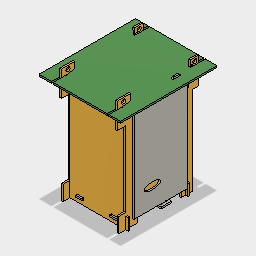
shelter2018-03 (Autodesk Fusion 360 design; units mm, degrees)
Autodesk Fusion 360 part; units mm, degrees
note: some values were not read from the file. Chosen so that the rebuilt part matches the saved one: which face or edge a step refers to. Set by a fixed rule: which sketch regions a step uses.
(part 1 of 2)
sketch "Sketch1" plane through (0, 0, 0) normal (0, 1, 0) x (1, 0, 0)
sketch "Sketch2" plane through (0, 0, 0) normal (0, 1, 0) x (1, 0, 0)
  line L0 (-64.6444, 10.108) -> (17.9056, 10.108)
  line L1 (17.9056, 10.108) -> (17.9056, -78.792)
  line L2 (17.9056, -78.792) -> (-57.0244, -78.792)
  line L3 (-64.6444, -71.172) -> (-64.6444, 10.108)
  line L4 (-53.4684, -78.792) -> (-43.3084, -78.792)
  line L5 (-43.3084, -78.792) -> (-43.3084, -83.872)
  line L6 (-43.3084, -83.872) -> (-53.4684, -83.872)
  line L7 (-53.4684, -83.872) -> (-53.4684, -78.792)
  line L8 (-1.3984, -78.792) -> (10.7936, -78.792)
  line L9 (10.7936, -78.792) -> (10.7936, -83.872)
  line L10 (10.7936, -83.872) -> (-1.3984, -83.872)
  line L11 (-1.3984, -83.872) -> (-1.3984, -78.792)
  line L12 (-49.4044, 10.108) -> (-39.2444, 10.108)
  line L13 (-39.2444, 10.108) -> (-39.2444, 15.188)
  line L14 (-39.2444, 15.188) -> (-49.4044, 15.188)
  line L15 (-49.4044, 15.188) -> (-49.4044, 10.108)
  line L16 (-3.4304, 10.108) -> (9.7776, 10.108)
  line L17 (9.7776, 10.108) -> (9.7776, 15.188)
  line L18 (9.7776, 15.188) -> (-3.4304, 15.188)
  line L19 (-3.4304, 15.188) -> (-3.4304, 10.108)
  line L20 (17.9056, -18.467) -> (27.6846, -18.467)
  line L21 (27.6846, -18.467) -> (27.6846, -34.215)
  line L22 (27.6846, -34.215) -> (17.9056, -34.215)
  line L23 (17.9056, -34.215) -> (17.9056, -18.467)
  line L24 (20.6996, -22.785) -> (23.8746, -22.785)
  line L25 (23.8746, -22.785) -> (23.8746, -29.897)
  line L26 (23.8746, -29.897) -> (20.6996, -29.897)
  line L27 (20.6996, -29.897) -> (20.6996, -22.785)
  line L28 (-56.5164, -21.642) -> (-45.3404, -21.642)
  line L29 (-45.3404, -21.642) -> (-45.3404, -24.182)
  line L30 (-45.3404, -24.182) -> (-56.5164, -24.182)
  line L31 (-56.5164, -24.182) -> (-56.5164, -21.642)
  line L32 (-20.7024, -21.642) -> (-12.5744, -21.642)
  line L33 (-12.5744, -21.642) -> (-12.5744, -24.182)
  line L34 (-12.5744, -24.182) -> (-20.7024, -24.182)
  line L35 (-20.7024, -24.182) -> (-20.7024, -21.642)
  arc A0 (-64.6444, -71.172) -> (-57.0244, -78.792) centre (-57.0244, -71.172) ccw
  line L36 (-2.54, 5.08) -> (12.7, 5.08)
  line L37 (12.7, 5.08) -> (12.7, 0)
  line L38 (12.7, 0) -> (-2.54, 0)
  line L39 (-2.54, 0) -> (-2.54, 5.08)
  dimension "d13" = 2.54
  dimension "d14" = 2.54
  dimension "d15" = 3.175
  dimension "d16" = 2.794
  dimension "d17" = 88.9
  dimension "d18" = 3.81
  dimension "d19" = 5.08
  dimension "d20" = 5.08
  dimension "d21" = 82.55
  dimension "d22" = 11.176
  dimension "d24" = 10.16
  dimension "d25" = 12.192
  dimension "d26" = 7.112
  dimension "d27" = 11.176
  dimension "d28" = 8.128
  dimension "d29" = 30.48
  dimension "d30" = 8.128
  dimension "d31" = 10.16
  dimension "d32" = 15.24
  dimension "d33" = 13.208
  dimension "d34" = 8.128
  dimension "d36" = 31.75
  dimension "d37" = 28.575
  dimension "d38" = 4.318
  dimension "d39" = 4.318
  dimension "d40" = 7.112
  measures "d13" distance of L28.end L29.end
  measures "d14" distance of L32.end L33.end
  measures "d15" distance of L25.end L26.end
  measures "d16" distance of L23 L27
  measures "d17" distance of L0.end L1.end
  measures "d18" distance of L21 L25
  measures "d19" distance of L8.start L10.end
  measures "d20" distance of L16.start L18.end
  measures "d21" distance of L0.start L0.end
  measures "d22" distance of L3 L7
  measures "d24" distance of L5.end L6.end
  measures "d25" distance of L9.end L10.end
  measures "d26" distance of L1 L9
  measures "d27" distance of L29.end L30.end
  measures "d28" distance of L33.end L34.end
  measures "d29" distance of L1 L33
  measures "d30" distance of L3 L31
  measures "d31" distance of L13.end L14.end
  measures "d32" distance of L3 L15
  measures "d33" distance of L17.end L18.end
  measures "d34" distance of L1 L17
  measures "d36" distance of L0 L32
  measures "d37" distance of L0 L20
  measures "d38" distance of L20 L24
  measures "d39" distance of L22 L26
  measures "d40" distance of L24.end L25.end
extrude "Extrude4" add sketch "Sketch2" against normal blind 2.54 contours L0 L1 L2 L3 L4 L8 L12 L16 L23 A0 | L0 L12 L13 L14 L15 | L0 L16 L17 L18 L19 | L2 L4 L5 L6 L7 | L2 L8 L9 L10 L11 | L1 L20 L21 L22 L23 | L36 L37 L38 L39 makes body 1
sketch "Sketch1 (2)" plane through (0, 0, 78.792) normal (0, 0, 1) x (1, 0, 0) in component "front"
  line L0 (-1.3984, 0) -> (-43.3084, 0)
  line L1 (-43.3084, 0) -> (-43.3084, -2.54)
  line L2 (-43.3084, -2.54) -> (-1.3984, -2.54)
  line L3 (-1.3984, -2.54) -> (-1.3984, 0)
  line L4 (-56.5164, 0) -> (-45.3404, 0)
  line L5 (-45.3404, 0) -> (-56.5164, 0)
  line L6 (-20.7024, 0) -> (-12.5744, 0)
  line L7 (-12.5744, 0) -> (-20.7024, 0)
  line L8 (-3.4304, 0) -> (-39.2444, 0)
  line L9 (-39.2444, 0) -> (-49.4044, 0)
  line L10 (-49.4044, 0) -> (-64.6444, 0)
  line L11 (-57.0244, 0) -> (-64.6444, 0)
  line L12 (-57.0244, 0) -> (-53.4684, 0)
  line L13 (-53.4684, 0) -> (-43.3084, 0)
  line L14 (-43.3084, 0) -> (-1.3984, 0)
  line L15 (-1.3984, 0) -> (10.7936, 0)
  line L16 (10.7936, 0) -> (17.9056, 0)
  line L17 (17.9056, 0) -> (9.7776, 0)
  line L18 (9.7776, 0) -> (-3.4304, 0)
  line L19 (-64.6444, 152.4) -> (17.9056, 152.4)
  line L20 (17.9056, 152.4) -> (17.9056, -10.16)
  line L21 (17.9056, -10.16) -> (-64.6444, -10.16)
  line L22 (-64.6444, -10.16) -> (-64.6444, 152.4)
  line L23 (-53.4684, 0) -> (-53.4684, -2.54)
  line L24 (-43.3084, 0) -> (-53.4684, 0)
  line L25 (-43.3084, -2.54) -> (-53.4684, -2.54)
  line L26 (-43.3084, 0) -> (-43.3084, -2.54)
  line L27 (-1.3984, 0) -> (-1.3984, -2.54)
  line L28 (10.7936, 0) -> (-1.3984, 0)
  line L29 (10.7936, -2.54) -> (-1.3984, -2.54)
  line L30 (10.7936, 0) -> (10.7936, -2.54)
  line L31 (-64.6444, -10.16) -> (-71.12, -10.16)
  line L32 (-71.12, -10.16) -> (-71.12, 7.6202)
  line L33 (-71.12, 7.6202) -> (-64.6444, 7.6202)
  line L34 (-64.6444, 7.6202) -> (-64.6444, -10.16)
  line L35 (17.9056, 12.7) -> (17.9056, -10.16)
  line L36 (-68.5808, 144.7274) -> (-68.5808, 138.684)
  line L37 (-68.5808, 138.684) -> (-64.6444, 138.684)
  line L38 (-64.6444, 138.684) -> (-64.6444, 144.78)
  line L39 (-64.6444, -2.54) -> (-67.1844, -2.54)
  line L40 (-67.1844, -2.54) -> (-67.1844, 0)
  line L41 (-67.1844, 0) -> (-64.6444, 0)
  line L42 (-64.6444, 0) -> (-64.6444, -2.54)
  line L43 (-67.1844, 0) -> (-64.6444, 0)
  line L44 (-64.6444, 0) -> (-64.6444, 7.6202)
  line L45 (-64.6444, 7.6202) -> (-67.1844, 7.6202)
  line L46 (-68.5808, 138.684) -> (-64.6444, -2.54)
  line L47 (-67.1844, -2.54) -> (-67.4676, 7.6202)
  arc A0 (-64.6444, 144.78) -> (-68.5808, 144.7274) centre (-64.6444, -2.54) ccw
  line L48 (-23.3694, -10.16) -> (-23.3694, 152.4)
  line L49 (17.9056, 138.684) -> (17.9056, 144.78)
  line L50 (21.842, 144.7274) -> (21.842, 138.684)
  arc A1 (21.842, 144.7274) -> (17.9056, 144.78) centre (17.9056, -2.54) ccw
  line L51 (21.842, 138.684) -> (17.9056, 138.684)
  line L52 (20.4456, -2.54) -> (20.4456, 0)
  line L53 (17.9056, 0) -> (17.9056, -2.54)
  line L54 (24.3812, -10.16) -> (24.3812, 7.6202)
  line L55 (17.9056, 0) -> (17.9056, 7.6202)
  line L56 (17.9056, -2.54) -> (20.4456, -2.54)
  line L57 (20.4456, -2.54) -> (20.7288, 7.6202)
  line L58 (17.9056, 7.6202) -> (20.4456, 7.6202)
  line L59 (17.9056, 7.6202) -> (17.9056, -10.16)
  line L60 (24.3812, 7.6202) -> (17.9056, 7.6202)
  line L61 (20.4456, 0) -> (17.9056, 0)
  line L62 (17.9056, -10.16) -> (24.3812, -10.16)
  line L63 (20.4456, 0) -> (17.9056, 0)
  point P0 (-43.3084, 0)
  point P1 (-1.3984, -2.54)
  point P2 (17.9056, 0)
  point P3 (10.7936, 0)
  point P4 (-1.3984, 0)
  point P5 (10.7936, -2.54)
  point P6 (-43.3084, -2.54)
  point P7 (17.9056, 0)
  point P8 (20.6996, 0)
  point P9 (23.8746, 0)
  point P10 (27.6846, 0)
  dimension "d46" = 152.4
  dimension "d50" = 2.54
  dimension "d51" = 2.54
  measures "d46" distance of P2 L19
  measures "d50" distance of L39.start L39.end
  measures "d51" distance of L39.end L40.end
extrude "Extrude1" add sketch "Sketch1 (2)" along normal blind 2.54 separate body contours L0 L2 L3 L6 L7 L8 L14 L18 L27 L48 | L0 L6 L7 L8 L14 L15 L16 L17 L18 L19 L20 L28 L35 L48 L49 L55 L59 | L2 L16 L17 L20 L21 L29 L30 L35 L48 L53 L59 | L2 L4 L5 L10 L11 L12 L21 L22 L23 L25 L34 L42 L48 | L0 L1 L2 L8 L9 L14 L26 L48 | L0 L4 L5 L8 L9 L10 L11 L12 L13 L14 L19 L22 L24 L34 L38 L44 L48 | L20 L35 L54 L56 L57 L59 L60 L62 | L22 L31 L32 L33 L34 L39 L47 | L22 L36 L37 L38 A0 | L20 L49 L50 A1 L51 makes body 2 in component "front"
sketch "Sketch1 (3)" plane through (0, 0, -10.108) normal (0, 0, -1) x (-1, 0, 0) in component "back"
  line L0 (39.2444, 0) -> (3.4304, 0)
  line L1 (3.4304, 0) -> (3.4304, -2.54)
  line L2 (3.4304, -2.54) -> (39.2444, -2.54)
  line L3 (39.2444, -2.54) -> (39.2444, 0)
  line L4 (-9.7776, 0) -> (-17.9056, 0)
  line L5 (-17.9056, 0) -> (-17.9056, -2.54)
  line L6 (-17.9056, -2.54) -> (-9.7776, -2.54)
  line L7 (-9.7776, -2.54) -> (-9.7776, 0)
  line L8 (3.4304, -2.54) -> (3.4304, 0)
  line L9 (39.2444, 0) -> (3.4304, 0)
  line L10 (49.4044, 0) -> (39.2444, 0)
  line L11 (64.6444, 0) -> (49.4044, 0)
  line L12 (64.6444, -2.54) -> (64.6444, 0)
  line L13 (49.4044, -2.54) -> (64.6444, -2.54)
  line L14 (49.4044, -2.54) -> (49.4044, 0)
  line L15 (3.4304, -2.54) -> (39.2444, -2.54)
  line L16 (-9.7776, -2.54) -> (3.4304, -2.54)
  line L17 (-9.7776, 0) -> (-9.7776, -2.54)
  line L18 (-9.7776, 0) -> (-17.9056, 0)
  line L19 (-17.9056, 0) -> (-17.9056, -2.54)
  line L20 (-17.9056, -2.54) -> (-9.7776, -2.54)
  line L21 (3.4304, 0) -> (-9.7776, 0)
  line L22 (39.2444, 0) -> (39.2444, -2.54)
  line L23 (39.2444, -2.54) -> (49.4044, -2.54)
  line L24 (-17.9056, 0) -> (64.6444, 0)
  line L25 (64.6444, 0) -> (64.6444, 152.4)
  line L26 (64.6444, 152.4) -> (-17.9056, 152.4)
  line L27 (-17.9056, 152.4) -> (-17.9056, 0)
  line L28 (-17.9056, -2.54) -> (-20.4456, -2.54)
  line L29 (-20.4456, -2.54) -> (-20.7288, 7.6202)
  line L30 (-24.3812, 7.6202) -> (-20.7288, 7.6202)
  line L31 (-24.3812, -10.16) -> (-24.3812, 7.6202)
  line L32 (-24.3812, -10.16) -> (71.12, -10.16)
  line L33 (71.12, -10.16) -> (71.12, 7.6202)
  line L34 (71.12, 7.6202) -> (67.4676, 7.6202)
  line L35 (67.1844, -2.54) -> (67.4676, 7.6202)
  line L36 (64.6444, -2.54) -> (67.1844, -2.54)
  line L37 (23.3694, 152.4) -> (23.3694, 0)
  line L38 (-17.9056, 132.4457) -> (-22.9856, 132.4457)
  line L39 (-22.9856, 132.4457) -> (-22.9856, 144.7757)
  arc A0 (-17.9056, 144.8633) -> (-22.9856, 144.7757) centre (-17.9056, -2.54) ccw
  arc A1 (69.7244, 144.7757) -> (64.6444, 144.8633) centre (64.6444, -2.54) ccw
  line L40 (69.7244, 132.4457) -> (69.7244, 144.7757)
  line L41 (64.6444, 132.4457) -> (69.7244, 132.4457)
  point P0 (64.6444, -2.54)
  dimension "d54" = 152.4
  dimension "d55" = 5.08
  measures "d54" distance of L4.end L26.end
  measures "d55" distance of L27 L39
extrude "Extrude1'" add sketch "Sketch1 (3)" along normal blind 2.54 separate body contours L0 L1 L2 L3 L8 L9 L15 L22 L24 | L0 L9 L10 L11 L24 L25 L26 L37 | L0 L4 L9 L18 L21 L24 L26 L27 L37 | L2 L6 L13 L15 L16 L20 L23 L28 L29 L30 L31 L32 L33 L34 L35 L36 | L11 L12 L13 L14 L24 | L4 L5 L6 L7 L17 L18 L19 L20 L24 | L25 A1 L40 L41 | L27 L38 L39 A0 makes body 3 in component "back"
sketch "Sketch1 (4)" plane through (0, 0, 21.642) normal (0, 0, 1) x (1, 0, 0) in component "midwall"
  line L0 (-12.5744, 0) -> (-20.7024, 0)
  line L1 (-20.7024, 0) -> (-20.7024, -2.54)
  line L2 (-20.7024, -2.54) -> (-12.5744, -2.54)
  line L3 (-12.5744, -2.54) -> (-12.5744, 0)
  line L4 (27.6846, -2.54) -> (27.6846, 0)
  line L5 (27.6846, 0) -> (-12.5744, 0)
  line L6 (-12.5744, 0) -> (-12.5744, -2.54)
  line L7 (-20.7024, -2.54) -> (-12.5744, -2.54)
  line L8 (-20.7024, -2.54) -> (-20.7024, 0)
  line L9 (-20.7024, 0) -> (-45.3404, 0)
  line L10 (-45.3404, 0) -> (-45.3404, -2.54)
  line L11 (-56.5164, -2.54) -> (-45.3404, -2.54)
  line L12 (-56.5164, -2.54) -> (-56.5164, 0)
  line L13 (-56.5164, 0) -> (-64.6444, 0)
  line L14 (-64.6444, 0) -> (-64.6444, -2.54)
  line L15 (-64.6444, -2.54) -> (-56.5164, -2.54)
  line L16 (-12.5744, -2.54) -> (27.6846, -2.54)
  line L17 (-12.5744, 0) -> (-20.7024, 0)
  line L18 (-45.3404, -2.54) -> (-20.7024, -2.54)
  line L19 (-45.3404, 0) -> (-56.5164, 0)
  line L20 (-64.6444, 0) -> (17.9056, 0)
  line L21 (17.9056, 0) -> (17.9056, 152.4)
  line L22 (17.9056, 152.4) -> (-64.6444, 152.4)
  line L23 (-64.6444, 152.4) -> (-64.6444, 0)
  line L24 (-53.2112, 152.4) -> (5.08, 152.4)
  line L25 (5.08, 152.4) -> (5.08, 139.7)
  line L26 (5.08, 139.7) -> (-53.2112, 139.7)
  line L27 (-53.2112, 139.7) -> (-53.2112, 152.4)
  line L28 (17.9056, 152.4) -> (20.6996, 152.4)
  line L29 (20.6996, 152.4) -> (20.6996, 145.288)
  line L30 (20.6996, 145.288) -> (17.9056, 145.288)
  line L31 (17.9056, 145.288) -> (17.9056, 152.4)
  line L32 (-64.6444, 152.4) -> (-69.7244, 152.4)
  line L33 (-69.7244, 152.4) -> (-69.7244, 145.288)
  line L34 (-69.7244, 145.288) -> (-64.6444, 145.288)
  line L35 (-64.6444, 145.288) -> (-64.6444, 152.4)
  line L36 (-51.9444, 114.3) -> (14.0956, 114.3)
  line L37 (14.0956, 114.3) -> (14.0956, 68.58)
  line L38 (14.0956, 68.58) -> (-51.9444, 68.58)
  line L39 (-51.9444, 68.58) -> (-51.9444, 114.3)
  line L40 (-39.2444, 19.05) -> (10.2856, 19.05)
  line L41 (10.2856, 19.05) -> (10.2856, 27.94)
  line L42 (10.2856, 27.94) -> (-39.2444, 27.94)
  line L43 (-39.2444, 27.94) -> (-39.2444, 19.05)
  circle A0 centre (-39.2444, 19.05) radius 1.27
  circle A1 centre (10.2856, 19.05) radius 1.27
  circle A2 centre (-51.9444, 68.58) radius 1.27
  circle A3 centre (14.0956, 68.58) radius 1.27
  circle A4 centre (14.0956, 114.3) radius 1.27
  circle A5 centre (-51.9444, 114.3) radius 1.27
  line L44 (-56.5164, 0) -> (-45.3404, 0)
  line L45 (-45.3404, 0) -> (-45.3404, -2.54)
  line L46 (-45.3404, -2.54) -> (-56.5164, -2.54)
  line L47 (-56.5164, -2.54) -> (-56.5164, 0)
  dimension "d58" = 82.55
  dimension "d59" = 152.4
  dimension "d60" = 2.794
  dimension "d61" = 5.08
  dimension "d62" = 7.112
  dimension "d68" = 3.81
  dimension "d69" = 45.72
  dimension "d70" = 66.04
  dimension "d71" = 25.4
  dimension "d72" = 49.53
  dimension "d75" = 19.05
  dimension "d76" = 2.54
  dimension "d77" = 2.54
  dimension "d78" = 2.54
  dimension "d79" = 2.54
  dimension "d80" = 2.54
  dimension "d81" = 2.54
  measures "d58" distance of L21.end L22.end
  measures "d59" distance of L20.end L21.end
  measures "d60" distance of L21.end L28.end
  measures "d61" distance of L22.end L32.end
  measures "d62" distance of L28.end L29.end
  measures "d68" distance of L21 L37
  measures "d69" distance of L36.end L37.end
  measures "d70" distance of L36.start L36.end
  measures "d71" distance of L23 L43
  measures "d72" distance of L41.end L42.end
  measures "d75" distance of L20 L40
  measures "d76" diameter of A5
  measures "d77" diameter of A4
  measures "d78" diameter of A2
  measures "d79" diameter of A3
  measures "d80" diameter of A0
  measures "d81" diameter of A1
extrude "Extrude1''" add sketch "Sketch1 (4)" along normal blind 2.54 separate body contours L0 L1 L2 L3 L6 L7 L8 L17 L20 | L0 L5 L9 L13 L17 L19 L20 L21 L22 L23 L25 L26 L27 L31 L35 L44 | L10 L11 L12 L19 L20 L44 L45 L46 L47 | L21 L28 L29 L30 L31 | L23 L32 L33 L34 L35 | L36 L37 L38 L39 A2 A3 A4 A5 | L40 L41 L42 L43 A0 A1 makes body 4 in component "midwall"
sketch "Sketch3" plane through (0, 0, 0) normal (0, 1, 0) x (1, 0, 0)
  line L0 (-39.2444, -24.182) -> (10.2856, -24.182)
  line L1 (10.2856, -24.182) -> (10.2856, -45.264)
  line L2 (10.2856, -45.264) -> (-39.2444, -45.264)
  line L3 (-39.2444, -45.264) -> (-39.2444, -24.182)
  line L4 (-64.6444, -71.172) -> (-64.6444, 10.108)
  line L5 (-7.2404, -27.484) -> (6.9836, -27.484)
  line L6 (6.9836, -27.484) -> (6.9836, -24.436)
  line L7 (6.9836, -24.436) -> (-7.2404, -24.436)
  line L8 (-7.2404, -24.436) -> (-7.2404, -27.484)
  line L9 (-39.2444, -34.723) -> (10.2856, -34.723)
  circle A0 centre (-25.0204, -34.723) radius 8.73
  line L10 (-12.5744, -24.182) -> (-20.7024, -24.182)
  dimension "d82" = 25.4
  dimension "d83" = 49.53
  dimension "d91" = 21.082
  dimension "d92" = 17.46
  dimension "d93" = 14.224
  dimension "d94" = 14.224
  dimension "d95" = 3.302
  dimension "d96" = 0.254
  dimension "d97" = 3.048
  measures "d82" distance of L3 L4
  measures "d83" distance of L1.end L2.end
  measures "d91" distance of L0.end L1.end
  measures "d92" diameter of A0
  measures "d93" distance of L3 A0.centre
  measures "d94" distance of L6.end L7.end
  measures "d95" distance of L1 L6
  measures "d96" distance of L0 L7
  measures "d97" distance of L5.start L7.end
extrude "Extrude6" cut sketch "Sketch2" sketch "Sketch3" against normal blind 2.54 contours L36 L37 L38 L39 of sketch 2 contours L9 A0 | L9 A0 | L5 L6 L7 L8 bodies 1
sketch "Sketch1 (5)" plane through (-64.6444, 0, 0) normal (-1, 0, 0) x (0, 0, 1) in component "left"
  line L0 (-10.108, -2.54) -> (-10.108, 132.4457)
  line L1 (-10.108, 132.4457) -> (-12.648, 132.4457)
  line L2 (-12.648, 132.4457) -> (-12.648, -2.54)
  line L3 (-12.648, -2.54) -> (-10.108, -2.54)
  line L4 (-12.648, 152.4) -> (81.332, 152.4)
  line L5 (81.332, 152.4) -> (81.332, -2.54)
  line L6 (81.332, -2.54) -> (-12.648, -2.54)
  line L7 (-12.648, -2.54) -> (-12.648, 152.4)
  line L8 (-10.108, -2.54) -> (-10.108, 132.4457)
  line L9 (-12.648, 132.4457) -> (-10.108, 132.4457)
  line L10 (-10.108, -2.54) -> (-10.108, 132.4457)
  line L11 (-10.108, -10.16) -> (-10.108, -2.54)
  line L12 (-12.648, -10.16) -> (-10.108, -10.16)
  line L13 (-12.648, -2.54) -> (-12.648, -10.16)
  line L14 (-10.108, -2.54) -> (-12.648, -2.54)
  line L15 (-12.648, 132.4457) -> (-12.648, -2.54)
  line L16 (-12.648, 144.8633) -> (-12.648, 132.4457)
  line L17 (-10.108, 144.8633) -> (-12.648, 144.8633)
  line L18 (-10.108, 144.8633) -> (-10.108, 152.4)
  line L19 (-10.108, 152.4) -> (-12.648, 152.4)
  line L20 (-12.648, 152.4) -> (-12.648, 144.8633)
  line L21 (-10.108, 132.4457) -> (-10.108, 144.8633)
  line L22 (24.182, 152.4) -> (21.642, 152.4)
  line L23 (21.642, 152.4) -> (21.642, 145.288)
  line L24 (21.642, 145.288) -> (24.182, 145.288)
  line L25 (24.182, 0) -> (24.182, 145.288)
  line L26 (21.642, 0) -> (24.182, 0)
  line L27 (21.642, 145.288) -> (21.642, 0)
  line L28 (24.182, 145.288) -> (24.182, 152.4)
  line L29 (78.792, -10.16) -> (81.332, -10.16)
  line L30 (81.332, -10.16) -> (81.332, -2.54)
  line L31 (81.332, -2.54) -> (78.792, -2.54)
  line L32 (78.792, 138.684) -> (78.792, -2.54)
  line L33 (78.792, 138.684) -> (81.332, 138.684)
  line L34 (81.332, 138.684) -> (81.332, 144.78)
  line L35 (81.332, 144.78) -> (78.792, 144.78)
  line L36 (78.792, 152.4) -> (78.792, 144.78)
  line L37 (81.332, 152.4) -> (78.792, 152.4)
  line L38 (81.332, 144.78) -> (81.332, 152.4)
  line L39 (78.792, -2.54) -> (78.792, -10.16)
  line L40 (81.332, -2.54) -> (81.332, 138.684)
  line L41 (78.792, 144.78) -> (78.792, 138.684)
  line L42 (71.172, -2.54) -> (-10.108, -2.54)
  line L43 (-3.4968, -2.54) -> (-12.648, -2.54)
  line L44 (-12.648, -2.54) -> (-12.648, -10.16)
  line L45 (-12.648, -10.16) -> (-3.4968, -10.16)
  line L46 (-3.4968, -10.16) -> (-3.4968, -2.54)
  line L47 (-12.648, -10.16) -> (-20.32, -10.16)
  line L48 (-20.32, -10.16) -> (-20.32, 10.16)
  line L49 (-20.32, 10.16) -> (-12.648, 10.16)
  line L50 (-12.648, 10.16) -> (-12.648, -10.16)
  line L51 (78.792, -10.16) -> (63.5, -10.16)
  line L52 (63.5, -10.16) -> (63.5, -2.54)
  line L53 (63.5, -2.54) -> (78.792, -2.54)
  line L54 (78.792, -2.54) -> (78.792, -10.16)
  line L55 (81.332, -10.16) -> (91.44, -10.16)
  line L56 (91.44, -10.16) -> (91.44, 12.7)
  line L57 (91.44, 12.7) -> (81.332, 12.7)
  line L58 (81.332, 12.7) -> (81.332, -10.16)
  line L59 (-12.648, 124.46) -> (-30.428, 124.46)
  line L60 (-30.428, 124.46) -> (-30.428, 152.4)
  line L61 (-30.428, 152.4) -> (-12.648, 152.4)
  line L62 (-12.648, 152.4) -> (-12.648, 124.46)
  line L63 (-30.428, 152.4) -> (-12.648, 152.4)
  line L64 (-17.1965, 165.1009) -> (-30.428, 165.1009)
  line L65 (-30.428, 165.1009) -> (-30.428, 152.4)
  line L66 (81.332, 127.3528) -> (94.032, 127.3528)
  line L67 (94.032, 127.3528) -> (94.032, 152.4009)
  line L68 (94.032, 152.4009) -> (81.332, 152.4009)
  line L69 (81.332, 152.4009) -> (81.332, 127.3528)
  line L70 (94.032, 152.4009) -> (86.7309, 152.4009)
  line L71 (78.74, 155.9553) -> (78.74, 166.37)
  line L72 (78.74, 166.37) -> (94.032, 166.37)
  line L73 (94.032, 166.37) -> (94.032, 152.4009)
  line L74 (78.74, 166.37) -> (73.712, 166.37)
  line L75 (73.712, 152.4) -> (85.5242, 152.4)
  line L76 (78.74, 155.9553) -> (78.74, 166.37)
  line L77 (-12.648, 152.4) -> (-17.1965, 152.4)
  line L78 (-17.1965, 152.4) -> (-17.1965, 165.1009)
  line L79 (-17.1965, 165.1009) -> (86.7309, 152.4009)
  line L80 (86.7309, 152.4009) -> (87.0413, 154.9409)
  line L81 (87.0413, 154.9409) -> (-16.8861, 167.6409)
  line L82 (-16.8861, 167.6409) -> (-17.1965, 165.1009)
  line L83 (73.712, 166.37) -> (73.712, 156.5697)
  line L84 (73.712, 153.9918) -> (73.712, 152.4)
  circle A0 centre (84.1517, 161.0274) radius 3.175
  circle A1 centre (-24.5119, 159.7522) radius 3.175
  circle A2 centre (-20.32, 156.21) radius 1.27
  arc A3 (-16.8861, 167.6409) -> (-18.014, 152.4) centre (85.5242, 152.4) ccw
  circle A4 centre (-21.6948, 142.2077) radius 3.175
  line L85 (81.332, -2.54) -> (81.332, 138.684)
  line L86 (-12.648, 144.7757) -> (-12.648, 132.4457)
  dimension "d100" = 2.54
  dimension "d101" = 6.35
  dimension "d103" = 6.35
  dimension "d104" = 2.54
  dimension "d105" = 6.35
  dimension "d143" = 20.32
  dimension "d144" = 12.7
  dimension "d145" = 13.97
  dimension "d146" = 27.94
  dimension "d147" = 17.78
  dimension "d177" = 3.81
  measures "d100" distance of L70.end L80.end
  measures "d101" diameter of A0
  measures "d103" diameter of A1
  measures "d104" diameter of A2
  measures "d105" diameter of A4
  measures "d143" distance of L73 L83
  measures "d144" distance of L67 L85
  measures "d145" distance of L74 L75
  measures "d146" distance of L59.end L60.end
  measures "d147" distance of L60 L86
  measures "d177" distance of L61 A2.centre
extrude "Extrude3" add sketch "Sketch1 (5)" along normal blind 2.54 separate body contours L0 L1 L2 L3 L6 L7 L8 L9 L10 L14 L15 L43 L50 L62 | L0 L4 L6 L8 L10 L18 L21 L23 L25 L26 L27 L28 L32 L36 L41 L42 L43 L53 L75 | L6 L11 L42 L43 L45 L46 | L2 L7 L13 L15 L44 L47 L48 L49 L50 | L2 L7 L15 L16 L20 L59 L60 L61 L62 L63 L77 L86 | L4 L7 L17 L18 L19 L20 L62 | L6 L39 L42 L51 L52 L53 L54 | L5 L6 L31 L32 L33 L40 L58 L69 L85 | L61 L63 L64 L65 A3 | L24 L25 L26 L27 | L5 L30 L40 L55 L56 L57 L58 L85 | L5 L34 L38 L40 L66 L67 L68 L69 L70 L75 L85 | L4 L5 L35 L36 L37 L38 L69 L75 | L68 L70 L71 L72 L73 L76 L80 L81 | L71 L74 L76 L81 L83 makes body 5 in component "left"
sketch "Sketch1 (6)" plane through (17.9056, 0, 0) normal (1, 0, 0) x (0, 0, -1) in component "right"
  line L0 (-78.792, -2.54) -> (-78.792, 138.684)
  line L1 (-78.792, 138.684) -> (-81.332, 138.684)
  line L2 (-81.332, 138.684) -> (-81.332, -2.54)
  line L3 (-81.332, -2.54) -> (-78.792, -2.54)
  line L4 (10.108, 144.8633) -> (12.648, 144.8633)
  line L5 (12.648, 144.8633) -> (12.648, 132.4457)
  line L6 (12.648, 132.4457) -> (10.108, 132.4457)
  line L7 (10.108, 132.4457) -> (10.108, 144.8633)
  circle A0 centre (21.6948, 142.2077) radius 3.175
  circle A1 centre (20.0726, 156.1629) radius 1.27
  line L8 (-81.332, 144.78) -> (-78.792, 144.78)
  line L9 (-78.792, 144.78) -> (-78.792, 138.684)
  line L10 (-78.792, 138.684) -> (-81.332, 138.684)
  line L11 (-81.332, 138.684) -> (-81.332, 144.78)
  line L12 (-73.712, 166.37) -> (-94.032, 166.37)
  line L13 (-94.032, 166.37) -> (-94.032, 127.3528)
  line L14 (-94.032, 127.3528) -> (-81.332, 127.3528)
  line L15 (-81.332, 127.3528) -> (-81.332, 12.7)
  line L16 (-81.332, 12.7) -> (-91.44, 12.7)
  line L17 (-91.44, 12.7) -> (-91.44, -10.16)
  line L18 (-91.44, -10.16) -> (-81.332, -10.16)
  line L19 (-81.332, -10.16) -> (-81.332, -2.54)
  line L20 (-81.332, -2.54) -> (-78.792, -2.54)
  line L21 (-78.792, -2.54) -> (-78.792, -10.16)
  line L22 (-78.792, -10.16) -> (-63.5, -10.16)
  line L23 (-63.5, -10.16) -> (-63.5, -2.54)
  line L24 (-63.5, -2.54) -> (3.4968, -2.54)
  line L25 (3.4968, -2.54) -> (3.4968, -10.16)
  line L26 (3.4968, -10.16) -> (10.108, -10.16)
  line L27 (10.108, -10.16) -> (10.108, -2.54)
  line L28 (10.108, -2.54) -> (12.648, -2.54)
  line L29 (12.648, -2.54) -> (12.648, -10.16)
  line L30 (12.648, -10.16) -> (20.32, -10.16)
  line L31 (20.32, -10.16) -> (20.32, 10.16)
  line L32 (20.32, 10.16) -> (12.648, 10.16)
  line L33 (12.648, 10.16) -> (12.648, 124.46)
  line L34 (12.648, 124.46) -> (30.428, 124.46)
  line L35 (30.428, 124.46) -> (30.428, 165.1009)
  line L36 (30.428, 165.1009) -> (17.232, 165.1009)
  arc A2 (18.014, 152.4) -> (17.232, 165.1009) centre (-85.5242, 152.4) ccw
  line L37 (18.014, 152.4) -> (17.1965, 152.4)
  line L38 (17.1965, 152.4) -> (-21.642, 152.4)
  line L39 (-21.642, 152.4) -> (-21.642, 145.288)
  line L40 (-21.642, 145.288) -> (-24.182, 145.288)
  line L41 (-24.182, 145.288) -> (-24.182, 152.4)
  line L42 (-24.182, 152.4) -> (-81.332, 152.4)
  line L43 (-86.7309, 152.4009) -> (-87.0413, 154.9409)
  line L44 (-87.0413, 154.9409) -> (-73.712, 156.5697)
  line L45 (-73.712, 156.5697) -> (-73.712, 166.37)
  line L46 (-21.642, 152.4) -> (10.108, 152.4)
  line L47 (10.108, 152.4) -> (10.108, -2.54)
  line L48 (10.108, -2.54) -> (-21.642, -2.54)
  line L49 (-12.752, 139.7) -> (-1.322, 139.7)
  line L50 (6.298, 132.08) -> (6.298, 13.97)
  line L51 (-1.322, 6.35) -> (-12.752, 6.35)
  line L52 (12.648, 124.46) -> (20.32, 124.46)
  line L53 (20.32, 124.46) -> (20.32, 10.16)
  line L54 (20.32, 10.16) -> (12.648, 10.16)
  line L55 (12.648, 10.16) -> (12.648, 124.46)
  line L56 (10.108, 0) -> (-78.792, 0)
  line L57 (-27.992, 120.65) -> (-41.962, 120.65)
  line L58 (-49.582, 113.03) -> (-49.582, 69.85)
  line L59 (-41.962, 62.23) -> (-27.992, 62.23)
  line L60 (-24.182, 0) -> (-24.182, 145.288)
  arc A3 (-12.752, 139.7) -> (-20.372, 132.08) centre (-12.752, 132.08) ccw
  arc A4 (6.298, 132.08) -> (-1.322, 139.7) centre (-1.322, 132.08) ccw
  arc A5 (-20.372, 13.97) -> (-12.752, 6.35) centre (-12.752, 13.97) ccw
  arc A6 (-1.322, 6.35) -> (6.298, 13.97) centre (-1.322, 13.97) ccw
  arc A7 (-49.582, 69.85) -> (-41.962, 62.23) centre (-41.962, 69.85) ccw
  arc A8 (-41.962, 120.65) -> (-49.582, 113.03) centre (-41.962, 113.03) ccw
  line L61 (-20.372, 13.97) -> (-20.372, 54.61)
  line L62 (-20.372, 128.27) -> (-20.372, 132.08)
  arc A9 (-27.992, 120.65) -> (-20.372, 128.27) centre (-27.992, 128.27) ccw
  line L63 (-21.642, -2.54) -> (-21.642, 0)
  line L64 (-21.642, 124.0579) -> (-21.642, 152.4)
  arc A10 (-20.372, 54.61) -> (-27.992, 62.23) centre (-27.992, 54.61) ccw
  circle A11 centre (24.5119, 159.7522) radius 3.175
  circle A12 centre (-84.1517, 161.0274) radius 3.175
  line L65 (-81.332, 152.4) -> (-81.332, 152.4009)
  line L66 (-81.332, 152.4009) -> (-86.7309, 152.4009)
  line L67 (-34.215, 0) -> (-34.215, -2.54)
  line L68 (-18.467, 0) -> (-18.467, -2.54)
  line L69 (-87.0413, 154.9409) -> (16.8861, 167.6409)
  circle A13 centre (20.32, 156.21) radius 1.27
  line L70 (-78.792, 138.684) -> (-78.792, 144.78)
  line L71 (-81.332, 138.684) -> (-78.792, 138.684)
  line L72 (-81.332, 144.78) -> (-81.332, 138.684)
  line L73 (-78.792, 144.78) -> (-81.332, 144.78)
  circle A14 centre (21.6948, 142.2077) radius 3.175
  circle A15 centre (-84.1517, 161.0274) radius 3.175
  circle A16 centre (24.5119, 159.7522) radius 3.175
  line L74 (10.108, 132.4457) -> (12.648, 132.4457)
  line L75 (10.108, 144.8633) -> (10.108, 132.4457)
  line L76 (12.648, 144.8633) -> (10.108, 144.8633)
  line L77 (12.648, 132.4457) -> (12.648, 144.8633)
  line L78 (-78.792, -2.54) -> (-81.332, -2.54)
  line L79 (-78.792, -10.16) -> (-78.792, -2.54)
  line L80 (-63.5, -10.16) -> (-78.792, -10.16)
  line L81 (-63.5, -2.54) -> (-63.5, -10.16)
  line L82 (3.4968, -2.54) -> (-63.5, -2.54)
  line L83 (3.4968, -10.16) -> (3.4968, -2.54)
  line L84 (10.108, -10.16) -> (3.4968, -10.16)
  line L85 (10.108, -2.54) -> (10.108, -10.16)
  line L86 (12.648, -2.54) -> (10.108, -2.54)
  line L87 (12.648, -10.16) -> (12.648, -2.54)
  line L88 (20.32, -10.16) -> (12.648, -10.16)
  line L89 (20.32, 10.16) -> (20.32, -10.16)
  line L90 (12.648, 10.16) -> (20.32, 10.16)
  line L91 (12.648, 124.46) -> (12.648, 10.16)
  line L92 (30.428, 124.46) -> (12.648, 124.46)
  line L93 (30.428, 165.1009) -> (30.428, 124.46)
  line L94 (17.232, 165.1009) -> (30.428, 165.1009)
  arc A17 (18.014, 152.4) -> (17.232, 165.1009) centre (-85.5242, 152.4) ccw
  line L95 (-21.642, 152.4) -> (18.014, 152.4)
  line L96 (-21.642, 145.288) -> (-21.642, 152.4)
  line L97 (-24.182, 145.288) -> (-21.642, 145.288)
  line L98 (-24.182, 152.4) -> (-24.182, 145.288)
  line L99 (-81.332, 152.4) -> (-24.182, 152.4)
  line L100 (-81.332, 152.4009) -> (-81.332, 152.4)
  line L101 (-86.7309, 152.4009) -> (-81.332, 152.4009)
  line L102 (-87.0413, 154.9409) -> (-86.7309, 152.4009)
  line L103 (-73.712, 156.5697) -> (-87.0413, 154.9409)
  line L104 (-73.712, 166.37) -> (-73.712, 156.5697)
  line L105 (-94.032, 166.37) -> (-73.712, 166.37)
  line L106 (-94.032, 127.3528) -> (-94.032, 166.37)
  line L107 (-81.332, 127.3528) -> (-94.032, 127.3528)
  line L108 (-81.332, 12.7) -> (-81.332, 127.3528)
  line L109 (-91.44, 12.7) -> (-81.332, 12.7)
  line L110 (-91.44, -10.16) -> (-91.44, 12.7)
  line L111 (-81.332, -10.16) -> (-91.44, -10.16)
  line L112 (-81.332, -2.54) -> (-81.332, -10.16)
  point P0 (-24.182, 68.58)
  point P1 (-24.182, 114.3)
  point P2 (-84.1517, 161.0274)
  dimension "d108" = 3.81
  dimension "d109" = 1.27
  dimension "d110" = 12.7
  dimension "d111" = 6.35
  dimension "d112" = 25.4
  dimension "d113" = 6.35
  dimension "d114" = 6.35
  dimension "d115" = 7.62
  dimension "d116" = 7.62
  dimension "d117" = 7.62
  dimension "d150" = 6.35
  measures "d108" distance of L47 L50
  measures "d109" distance of L61 L63
  measures "d110" distance of L46 L49
  measures "d111" distance of L51 L56
  measures "d112" distance of L58 L60
  measures "d113" distance of L57 P1
  measures "d114" distance of L59 P0
  measures "d115" radius of A3
  measures "d116" radius of A9
  measures "d117" radius of A10
  measures "d150" diameter of A12
extrude "Extrude3'" add sketch "Sketch1 (6)" along normal blind 2.54 separate body contours L0 L1 L2 L3 L10 L15 L20 L71 L78 L108 | L0 L21 L22 L23 L24 L56 L67 L79 L80 L81 L82 | L0 L2 L8 L9 L11 L12 L13 L14 L41 L42 L43 L44 L45 L56 L57 L58 L59 L60 A7 A8 A9 A10 L66 L69 L70 L72 L73 L98 L99 L101 L102 L103 L104 L105 L106 L107 | L2 L16 L17 L18 L19 L109 L110 L111 L112 | L7 L38 L39 L46 L47 L49 L50 L51 L56 L60 A3 A4 A5 A6 L61 L62 A9 L64 A10 L75 L95 L96 | L24 L47 L48 L56 L68 L82 | L40 L60 A9 L64 L97 | L4 L5 L6 L28 L29 L30 L31 L32 L33 L34 L35 L36 A2 L37 L38 L47 L52 L54 L55 L74 L76 L77 L86 L87 L88 L89 L90 L91 L92 L93 L94 A17 L95 | L25 L26 L27 L48 L83 L84 L85 | L32 L33 L34 L52 L53 L54 L55 L90 L91 L92 makes body 6 in component "right"
sketch "Sketch1 (7)" plane through (0, 152.4, 0) normal (0, 1, 0) x (-1, 0, 0) in component "top"
  line L0 (-17.9056, 24.182) -> (-17.9056, 81.332)
  line L1 (-17.9056, 81.332) -> (-20.4456, 81.332)
  line L2 (-20.4456, 81.332) -> (-20.4456, 24.182)
  line L3 (-20.4456, 24.182) -> (-17.9056, 24.182)
  line L4 (86.36, -40.64) -> (-38.1, -40.64)
  line L5 (-38.1, -40.64) -> (-38.1, 106.68)
  line L6 (-38.1, 106.68) -> (86.36, 106.68)
  line L7 (86.36, 106.68) -> (86.36, -40.64)
  line L8 (67.1844, 21.642) -> (64.6444, 21.642)
  line L9 (64.6444, 21.642) -> (64.6444, -18.014)
  line L10 (67.1844, -18.014) -> (64.6444, -18.014)
  line L11 (67.1844, -30.428) -> (67.1844, -18.014)
  line L12 (64.6444, -30.428) -> (67.1844, -30.428)
  line L13 (64.6444, -18.014) -> (64.6444, -30.428)
  line L14 (67.1844, -18.014) -> (67.1844, 21.642)
  line L15 (67.1844, 94.032) -> (64.6444, 94.032)
  line L16 (64.6444, 94.032) -> (64.6444, 81.332)
  line L17 (64.6444, 81.332) -> (67.1844, 81.332)
  line L18 (67.1844, 24.182) -> (67.1844, 81.332)
  line L19 (64.6444, 24.182) -> (67.1844, 24.182)
  line L20 (64.6444, 81.332) -> (64.6444, 24.182)
  line L21 (67.1844, 81.332) -> (67.1844, 94.032)
  line L22 (-20.4456, -30.428) -> (-17.9056, -30.428)
  line L23 (-17.9056, -30.428) -> (-17.9056, -18.014)
  line L24 (-17.9056, -18.014) -> (-20.4456, -18.014)
  line L25 (-20.4456, 21.642) -> (-20.4456, -18.014)
  line L26 (-17.9056, 21.642) -> (-20.4456, 21.642)
  line L27 (-17.9056, -18.014) -> (-17.9056, 21.642)
  line L28 (-20.4456, -18.014) -> (-20.4456, -30.428)
  line L29 (-20.4456, 24.182) -> (-17.9056, 24.182)
  line L30 (-17.9056, 24.182) -> (-17.9056, 81.332)
  line L31 (-20.4456, 81.332) -> (-17.9056, 81.332)
  line L32 (-20.4456, 94.032) -> (-20.4456, 81.332)
  line L33 (-17.9056, 94.032) -> (-20.4456, 94.032)
  line L34 (-17.9056, 81.332) -> (-17.9056, 94.032)
  line L35 (-20.4456, 81.332) -> (-20.4456, 24.182)
  line L36 (67.1844, 94.032) -> (64.6444, 94.032)
  line L37 (64.6444, 94.032) -> (64.6444, 106.68)
  line L38 (64.6444, 106.68) -> (67.1844, 106.68)
  line L39 (67.1844, 106.68) -> (67.1844, 94.032)
  line L40 (-17.9056, 94.032) -> (-20.4456, 94.032)
  line L41 (-20.4456, 94.032) -> (-20.4456, 106.68)
  line L42 (-20.4456, 106.68) -> (-17.9056, 106.68)
  line L43 (-17.9056, 106.68) -> (-17.9056, 94.032)
  line L44 (-20.4456, -30.428) -> (-17.9056, -30.428)
  line L45 (-17.9056, -30.428) -> (-17.9056, -40.64)
  line L46 (-17.9056, -40.64) -> (-20.4456, -40.64)
  line L47 (-20.4456, -40.64) -> (-20.4456, -30.428)
  line L48 (64.6444, -30.428) -> (67.1844, -30.428)
  line L49 (67.1844, -30.428) -> (67.1844, -40.64)
  line L50 (67.1844, -40.64) -> (64.6444, -40.64)
  line L51 (64.6444, -40.64) -> (64.6444, -30.428)
extrude "Extrude1'''" add sketch "Sketch1 (7)" along normal blind 2.54 separate body contours L0 L1 L2 L3 L29 L30 L31 L35 | L0 L2 L3 L4 L5 L6 L7 L8 L9 L11 L13 L14 L16 L18 L19 L20 L21 L23 L25 L26 L27 L28 L29 L30 L32 L34 L35 L37 L39 L41 L43 L45 L47 L49 L51 | L17 L18 L19 L20 | L24 L25 L26 L27 | L8 L9 L10 L14 makes body 7 in component "top"
sketch "Sketch1 (8)" plane through (20.6996, 0, 0) normal (1, 0, 0) x (0, 0, -1) in component "door (1)"
  line L0 (-22.785, 0) -> (-29.897, 0)
  line L1 (-29.897, 0) -> (-29.897, -2.54)
  line L2 (-29.897, -2.54) -> (-22.785, -2.54)
  line L3 (-22.785, -2.54) -> (-22.785, 0)
  line L4 (10.108, 152.4) -> (-71.172, 152.4)
  line L5 (-71.172, 152.4) -> (-71.172, 0)
  line L6 (-71.172, 0) -> (10.108, 0)
  line L7 (10.108, 0) -> (10.108, 152.4)
  line L8 (-71.172, 152.4) -> (10.108, 152.4)
  line L9 (10.108, 152.4) -> (10.108, 146.05)
  line L10 (10.108, 146.05) -> (-71.172, 146.05)
  line L11 (-71.172, 146.05) -> (-71.172, 152.4)
  line L12 (40.64, 152.4) -> (-106.68, 152.4)
  line L13 (10.108, 146.05) -> (-71.172, 139.3173)
  line L14 (-11.7805, 144.2369) -> (-0.3486, 144.2369)
  line L15 (-0.3486, 144.2369) -> (-0.3486, 154.94)
  line L16 (-0.3486, 154.94) -> (-11.7805, 154.94)
  line L17 (-11.7805, 154.94) -> (-11.7805, 144.2369)
  line L18 (40.64, 154.94) -> (-106.68, 154.94)
  line L19 (-0.3486, 154.94) -> (-11.7805, 154.94)
  line L20 (-11.7805, 154.94) -> (-11.7805, 155.448)
  line L21 (-9.7485, 157.48) -> (-2.3806, 157.48)
  line L22 (-0.3486, 155.448) -> (-0.3486, 154.94)
  line L23 (-106.68, 154.94) -> (40.64, 154.94)
  line L24 (-29.897, -2.54) -> (-22.785, -2.54)
  line L25 (-22.785, -2.54) -> (-22.785, -3.048)
  line L26 (-24.817, -5.08) -> (-27.865, -5.08)
  line L27 (-29.897, -3.048) -> (-29.897, -2.54)
  ellipse E0 centre (-43.18, 30.48) end of major axis (-55.88, 30.48) minor radius 5.1848
  line L28 (-30.48, 30.48) -> (-55.88, 30.48)
  line L29 (-43.18, 35.6648) -> (-43.18, 25.2952)
  arc A0 (-0.3486, 155.448) -> (-2.3806, 157.48) centre (-2.3806, 155.448) ccw
  arc A1 (-9.7485, 157.48) -> (-11.7805, 155.448) centre (-9.7485, 155.448) ccw
  arc A2 (-24.817, -5.08) -> (-22.785, -3.048) centre (-24.817, -3.048) ccw
  arc A3 (-29.897, -3.048) -> (-27.865, -5.08) centre (-27.865, -3.048) ccw
  point P0 (10.108, 152.4)
  point P1 (-71.172, 0)
  dimension "d159" = 6.35
  dimension "d160" = 2.54
  dimension "d161" = 2.54
  dimension "d162" = 2.032
  dimension "d163" = 2.032
  dimension "d164" = 2.032
  measures "d159" distance of L10 L12
  measures "d160" distance of L21 L23
  measures "d161" distance of L24 L26
  measures "d162" radius of A0
  measures "d163" radius of A1
  measures "d164" radius of A2
extrude "Extrude1''''" add sketch "Sketch1 (8)" along normal blind 2.54 separate body contours L0 L1 L2 L3 L6 L24 | L0 L5 L6 L7 L13 L14 L15 | L2 L24 L25 L26 L27 A2 A3 | L10 L13 L15 L17 | L4 L8 L10 L12 L15 L17 | L13 L14 L15 | L4 L8 L12 L15 L16 L17 L18 L19 L23 | L16 L18 L19 L20 L21 L22 L23 A0 A1 makes body 8 in component "door (1)"
sketch "Sketch2 (2)" plane through (0, 154.94, 0) normal (0, 1, 0) x (-1, 0, 0) in component "top"
  line L0 (-17.9056, -18.014) -> (-17.9056, -40.64)
  line L1 (-17.9056, -40.64) -> (64.6444, -40.64)
  line L2 (64.6444, -40.64) -> (64.6444, -18.014)
  line L3 (64.6444, -18.014) -> (67.1844, -18.014)
  line L4 (67.1844, -18.014) -> (67.1844, -40.64)
  line L5 (67.1844, -40.64) -> (86.36, -40.64)
  line L6 (86.36, -40.64) -> (86.36, 106.68)
  line L7 (86.36, 106.68) -> (67.1844, 106.68)
  line L8 (67.1844, 106.68) -> (67.1844, 81.332)
  line L9 (67.1844, 81.332) -> (64.6444, 81.332)
  line L10 (64.6444, 81.332) -> (64.6444, 106.68)
  line L11 (64.6444, 106.68) -> (-17.9056, 106.68)
  line L12 (-17.9056, 106.68) -> (-17.9056, 81.332)
  line L13 (-17.9056, 81.332) -> (-20.4456, 81.332)
  line L14 (-20.4456, 81.332) -> (-20.4456, 106.68)
  line L15 (-20.4456, 106.68) -> (-38.1, 106.68)
  line L16 (-38.1, 106.68) -> (-38.1, -40.64)
  line L17 (-38.1, -40.64) -> (-20.4456, -40.64)
  line L18 (-20.4456, -40.64) -> (-20.4456, -18.014)
  line L19 (-20.4456, -18.014) -> (-17.9056, -18.014)
  line L20 (-20.6996, 11.7805) -> (-23.2396, 11.7805)
  line L21 (-23.2396, 11.7805) -> (-23.2396, 0.3486)
  line L22 (-23.2396, 0.3486) -> (-20.6996, 0.3486)
  line L23 (-20.6996, 0.3486) -> (-20.6996, 11.7805)
extrude "Extrude2" cut sketch "Sketch2 (2)" against normal blind 2.54 contours L20 L21 L22 L23 bodies 7 in component "top"
extrude "Extrude1'''''" [suppressed] in component "right"
sketch "Sketch2 (3)" plane through (20.6996, 0, 0) normal (1, 0, 0) x (0, 0, -1) in component "door"
  line L0 (-22.785, 0) -> (-29.897, 0)
  line L1 (-29.897, 0) -> (-29.897, -2.54)
  line L2 (-29.897, -2.54) -> (-22.785, -2.54)
  line L3 (-22.785, -2.54) -> (-22.785, 0)
  line L4 (-29.897, 0) -> (-29.897, -2.54)
  line L5 (-22.785, 0) -> (-22.785, -2.54)
  line L6 (10.108, 0) -> (-78.792, 0)
  line L7 (-81.332, 127.3528) -> (-81.332, 12.7)
  line L8 (-24.182, 152.4) -> (-81.332, 152.4)
  line L9 (10.108, 132.4457) -> (10.108, 144.7757)
  line L10 (0, 0) -> (-62.282, 0)
  line L11 (-62.282, 0) -> (-62.282, 146.05)
  ellipse E0 centre (-42.3824, 40.1076) end of major axis (-29.6824, 40.1076) minor radius 5.1202
  line L12 (-55.0824, 40.1076) -> (-29.6824, 40.1076)
  line L13 (-42.3824, 34.9874) -> (-42.3824, 45.2277)
  line L14 (-49.582, 64.77) -> (-49.582, 113.03)
  line L15 (-62.282, 146.05) -> (8.838, 146.05)
  line L16 (8.838, 146.05) -> (8.838, 0)
  line L17 (8.838, 0) -> (-62.282, 0)
  line L18 (-62.282, 0) -> (-62.282, 146.05)
  line L19 (10.108, 132.4457) -> (10.108, -2.54)
  line L20 (-62.282, 135.89) -> (8.838, 146.05)
  line L21 (18.014, 152.4) -> (17.1965, 152.4)
  line L22 (17.1965, 152.4) -> (-21.642, 152.4)
  line L23 (18.014, 152.4) -> (17.1965, 152.4)
  line L24 (17.1965, 152.4) -> (-21.642, 152.4)
  line L25 (-10.6483, 143.2662) -> (-9.2397, 152.4)
  line L26 (-2.2228, 152.4) -> (-1.1126, 144.6285)
  line L27 (-9.2397, 152.4) -> (-8.4562, 157.48)
  line L28 (-8.4562, 157.48) -> (-2.9485, 157.48)
  line L29 (-2.9485, 157.48) -> (-2.2228, 152.4)
  line L30 (-29.897, 0) -> (-29.1242, -5.08)
  line L31 (-29.1242, -5.08) -> (-23.7323, -5.08)
  line L32 (-23.7323, -5.08) -> (-22.785, 0)
  line L33 (-9.2397, 152.4) -> (-2.9485, 152.4)
  line L34 (-2.9485, 152.4) -> (-2.9485, 157.48)
  line L35 (-2.9485, 157.48) -> (-9.2397, 157.48)
  line L36 (-9.2397, 157.48) -> (-9.2397, 152.4)
  line L37 (-2.2228, 152.4) -> (-2.9485, 152.4)
  line L38 (-2.9485, 152.4) -> (-2.9485, 157.48)
  line L39 (-2.9485, 157.48) -> (-2.2228, 157.48)
  line L40 (-2.2228, 157.48) -> (-2.2228, 152.4)
  point P0 (-22.785, 0)
  dimension "d120" = 12.7
  dimension "d121" = 1.27
  dimension "d122" = 10.16
  dimension "d123" = 6.35
  dimension "d133" = 5.08
  dimension "d134" = 5.08
  measures "d120" distance of L11 L14
  measures "d121" distance of L16 L19
  measures "d122" distance of L11.end L20.start
  measures "d123" distance of L15 L24
  measures "d133" distance of L22 L28
  measures "d134" distance of L10 L31
extrude "Extrude2'" [suppressed] in component "door"
sketch "Sketch1 (9)" plane through (0, 152.4, 0) normal (0, 1, 0) x (-1, 0, 0) in component "roof"
  line L0 (-17.9056, 24.182) -> (-17.9056, 81.332)
  line L1 (-20.4456, 81.332) -> (-20.4456, 24.182)
  line L2 (-20.4456, 24.182) -> (-17.9056, 24.182)
  line L3 (-20.4456, 24.182) -> (-17.9056, 24.182)
  line L4 (-17.9056, 24.182) -> (-17.9056, 81.332)
  line L5 (-20.4456, 94.032) -> (-20.4456, 81.332)
  line L6 (-17.9056, 94.032) -> (-20.4456, 94.032)
  line L7 (-17.9056, 81.332) -> (-17.9056, 94.032)
  line L8 (-20.4456, 81.332) -> (-20.4456, 24.182)
  line L9 (-17.9056, 21.642) -> (-20.4456, 21.642)
  line L10 (-20.4456, 21.642) -> (-20.4456, -17.1965)
  line L11 (-20.4456, -17.1965) -> (-20.4456, -18.014)
  line L12 (-17.9056, -18.014) -> (-20.4456, -18.014)
  line L13 (-17.9056, -30.428) -> (-17.9056, -18.014)
  line L14 (-20.4456, -30.428) -> (-17.9056, -30.428)
  line L15 (-20.4456, -18.014) -> (-20.4456, -30.428)
  line L16 (-17.9056, -17.1965) -> (-17.9056, 21.642)
  line L17 (-17.9056, -18.014) -> (-17.9056, -17.1965)
  line L18 (67.1844, 21.642) -> (64.6444, 21.642)
  line L19 (64.6444, 21.642) -> (64.6444, -17.2023)
  line L20 (64.6444, -17.2023) -> (64.6444, -18.014)
  line L21 (67.1844, -18.014) -> (64.6444, -18.014)
  line L22 (67.1844, -30.428) -> (67.1844, -18.014)
  line L23 (64.6444, -30.428) -> (67.1844, -30.428)
  line L24 (64.6444, -18.014) -> (64.6444, -30.428)
  line L25 (67.1844, -17.2023) -> (67.1844, 21.642)
  line L26 (67.1844, -18.014) -> (67.1844, -17.2023)
  line L27 (67.1844, 24.182) -> (67.1844, 81.332)
  line L28 (64.6444, 24.182) -> (67.1844, 24.182)
  line L29 (64.6444, 81.332) -> (64.6444, 24.182)
  line L30 (64.6444, 91.492) -> (64.6444, 86.7231)
  line L31 (67.1844, 91.492) -> (64.6444, 91.492)
  line L32 (67.1844, 86.7231) -> (67.1844, 91.492)
  line L33 (79.8844, -43.128) -> (79.8844, 106.732)
  line L34 (79.8844, 106.732) -> (-33.1456, 106.732)
  line L35 (-33.1456, 106.732) -> (-33.1456, -43.128)
  line L36 (-20.4456, -30.428) -> (-17.9056, -30.428)
  line L37 (-17.9056, -30.428) -> (-17.9056, -43.128)
  line L38 (-17.9056, -43.128) -> (-20.4456, -43.128)
  line L39 (-20.4456, -43.128) -> (-20.4456, -30.428)
  line L40 (64.6444, -30.428) -> (67.1844, -30.428)
  line L41 (67.1844, -30.428) -> (67.1844, -43.128)
  line L42 (67.1844, -43.128) -> (64.6444, -43.128)
  line L43 (64.6444, -43.128) -> (64.6444, -30.428)
  line L44 (64.6444, 91.492) -> (67.1844, 91.492)
  line L45 (67.1844, 91.492) -> (67.1844, 106.732)
  line L46 (67.1844, 106.732) -> (64.6444, 106.732)
  line L47 (64.6444, 106.732) -> (64.6444, 91.492)
  line L48 (-20.4456, 94.032) -> (-17.78, 94.032)
  line L49 (-17.78, 94.032) -> (-17.78, 106.732)
  line L50 (-17.78, 106.732) -> (-20.4456, 106.732)
  line L51 (-20.4456, 106.732) -> (-20.4456, 94.032)
  line L52 (-20.6996, -17.1965) -> (-20.6996, 21.642)
  line L53 (-23.2396, 2.5001) -> (-20.6996, 2.5001)
  line L54 (-20.6996, 2.5001) -> (-20.6996, 9.2397)
  line L55 (-20.6996, 9.2397) -> (-23.2396, 9.2397)
  line L56 (-23.2396, 9.2397) -> (-23.2396, 2.5001)
  line L57 (-23.4936, 5.08) -> (-23.2396, 5.08)
  line L58 (-20.6996, 5.08) -> (-20.4456, 5.08)
  line L59 (-33.1456, -43.128) -> (-17.9056, -43.128)
  line L60 (64.6444, -43.128) -> (79.8844, -43.128)
  line L61 (64.6444, -43.128) -> (-22.86, -43.128)
  line L62 (67.1844, 81.332) -> (64.6444, 81.332)
  line L63 (64.6444, 86.7231) -> (67.1844, 86.7231)
  line L64 (-17.9056, 81.332) -> (-20.4456, 81.332)
  line L65 (-20.4456, 81.332) -> (-17.9056, 81.332)
  dimension "d126" = 12.7
  dimension "d127" = 12.7
  dimension "d128" = 12.7
  dimension "d129" = 12.7
  measures "d126" distance of L32 L33
  measures "d127" distance of L5.start L35
  measures "d128" distance of L5.start L34
  measures "d129" distance of L13.start L59
extrude "Extrude3''" [suppressed] in component "roof"
copy_body "Body->Comp1" bodies 1 removing the originals makes body 10 in component "floorfromorig"
extrude "Extrude3'''" add 2 faces at (18.7523, 153.2467, 81.332) (-65.4911, 153.2467, 81.332) along direction (0, 0, 1) blind 5.08 on bodies 7 bodies 7 in component "top"